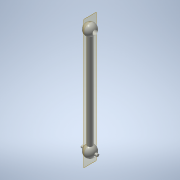
# Autodesk Inventor part: front_power_shaft
Saved by Autodesk Inventor 2020 (Build 240168000, 168)
## iProperties
Created: 2015-12-09
Part Number: front_power_shaft
Material: Genérico
Document SubType Name: Modeling
Designer: MIGUEL ANGEL
Density: 1 g/cm^3
Appearance: Suave - Marfil
Author: MIGUEL ANGEL
Autodesk Inventor part; units mm, degrees
ref_plane "XZ Plane" through (0, 0, 0) normal (0, 1, 0) x (-1, 0, 0)
sketch "Boceto1" plane through (0, 0, 0) normal (0, 0, 1) x (1, 0, 0)
  arc A0 (0, -9) -> (0, 9) centre (0, 0) ccw
  line L0 (0, 13.8048) -> (0, -12.2408)
  dimension "d0" = 18
  constraints: 2 end point, 2 point on circle, 2 point on line, 1 centre point, 1 coincident, 1 vertical
  measures "d0" diameter of A0
revolve "Revolución1" add sketch "Boceto1" angle 360 about axis through (0, 13.8048, 0) along (0, -1, 0)
sketch "Boceto2" plane through (0, 0, 0) normal (0, 0, 1) x (1, 0, 0)
  circle A0 centre (0, 0) radius 4
  dimension "d2" = 8
  constraints: 1 centre point, 1 coincident
  measures "d2" diameter of A0
extrude "Extrusión1" add sketch "Boceto2" along normal blind 165
ref_plane "Plano de trabajo1" through (0, 0, 82.5) normal (0, 0, 1) x (1, 0, 0)
mirror "Simetría1" about plane through (0, 0, 82.5) normal (0, 0, 1) of "Revolución1"
sketch "Boceto3" plane through (0, 0, 0) normal (1, 0, 0) x (0, 1, 0)
  circle A0 centre (0, 0) radius 2
  dimension "d5" = 4
  constraints: 1 centre point, 1 coincident
  measures "d5" diameter of A0
extrude "Extrusión2" add sketch "Boceto3" along normal mid plane 25
sketch "Boceto4" plane through (0, 0, 0) normal (1, 0, 0) x (0, 1, 0)
  arc A0 (4, 156.9377) -> (-4, 156.9377) centre (0, 165) ccw projected
  circle A1 centre (0, 165) radius 4
  point P0 (0, 0)
  dimension "d8" = 8
  dimension "d11" = 9
  constraints: 1 centre point, 1 coincident
  measures "d8" diameter of A1
  measures "d11" radius of A0
extrude "Extrusión3" cut sketch "Boceto4" along normal through all both and the other way through all
